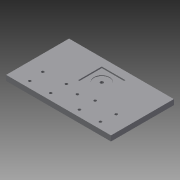
# Autodesk Inventor part: tractor
Saved by Autodesk Inventor 2013 (Build 170138000, 138)
## iProperties
Created: 2012-11-28
Part Number: tractor
Material: Generic
Document SubType Name: Modeling
Designer: Istvan
Density: 1 g/cm^3
Author: Istvan
Autodesk Inventor part; units mm, degrees
ref_plane "YZ Plane" through (0, 0, 0) normal (1, 0, 0) x (0, 1, 0)
ref_plane "XZ Plane" through (0, 0, 0) normal (0, 1, 0) x (-1, 0, 0)
ref_plane "XY Plane" through (0, 0, 0) normal (0, 0, 1) x (1, 0, 0)
sketch "Sketch1" plane through (0, 0, 0) normal (0, 1, 0) x (-1, 0, 0)
  line L0 (0, 0) -> (254, 0)
  line L1 (254, 0) -> (254, 152.4)
  line L2 (254, 152.4) -> (0, 152.4)
  line L3 (0, 152.4) -> (0, 0)
  dimension "d0" = 254
  dimension "d1" = 152.4
  constraints: 8 end point, 2 parallel, 1 horizontal, 1 perpendicular
  measures "d0" distance of L2.end L1.end
  measures "d1" distance of L1.end L0.end
extrude "Extrusion1" add sketch "Sketch1" against normal blind 12.7
sketch "Sketch2" plane through (0, 0, 0) normal (0, 1, 0) x (1, 0, 0)
  line L0 (0, 0) -> (-254, 0) projected
  line L1 (-254, 0) -> (-254, -152.4) projected
  line L2 (0, -152.4) -> (0, 0) projected
  line L3 (-155.575, -19.05) -> (-98.425, -19.05)
  line L4 (-98.425, -19.05) -> (-98.425, -76.2)
  line L5 (-98.425, -76.2) -> (-155.575, -76.2)
  line L6 (-155.575, -76.2) -> (-155.575, -19.05)
  dimension "d4" = 57.15
  dimension "d6" = 57.15
  dimension "d7" = 98.425
  dimension "d8" = 98.425
  dimension "d9" = 19.05
  constraints: 8 end point, 2 parallel, 1 horizontal, 1 perpendicular
  measures "d4" distance of L4.end L5.end
  measures "d6" distance of L3.end L4.end
  measures "d7" distance between parallel lines of L1 L6
  measures "d8" distance between parallel lines of L2 L4
  measures "d9" distance between parallel lines of L0 L3
extrude "Extrusion2" cut sketch "Sketch2" against normal blind 3.175
sketch "Sketch3" plane through (0, -3.175, 0) normal (0, 1, 0) x (1, 0, 0)
  line L0 (-98.425, -76.2) -> (-155.575, -76.2) projected
  line L1 (-98.425, -19.05) -> (-98.425, -76.2) projected
  circle A0 centre (-127, -47.625) radius 19.05
  point P0 (0, 0)
  dimension "d12" = 38.1
  dimension "d13" = 28.575
  dimension "d14" = 28.575
  constraints: 1 centre point
  measures "d12" diameter of A0
  measures "d13" distance from line of L0 A0.centre
  measures "d14" distance from line of L1 A0.centre
extrude "Extrusion3" cut sketch "Sketch3" against normal blind 1.524
sketch "Sketch4" plane through (-127, -4.699, 47.625) normal (0, 1, 0) x (1, 0, 0)
  circle A0 centre (0, 0) radius 19.05 projected
  circle A1 centre (0, 0) radius 3.81
  point P0 (127, 47.625)
  dimension "d17" = 7.62
  constraints: 1 centre point, 1 coincident
  measures "d17" diameter of A1
extrude "Extrusion4" cut sketch "Sketch4" against normal through all contours A1
sketch "Sketch5" plane through (0, -12.7, 0) normal (0, -1, 0) x (1, 0, 0)
  line L0 (0, 0) -> (0, 152.4) projected
  line L1 (0, 152.4) -> (-254, 152.4) projected
  line L2 (-254, 152.4) -> (-254, 0) projected
  circle A0 centre (-127, 47.625) radius 3.81 projected
  point P0 (-38.1, 101.6)
  point P1 (-215.9, 101.6)
  point P2 (-127, 106.68)
  dimension "d20" = 50.8
  dimension "d21" = 38.1
  dimension "d22" = 38.1
  dimension "d30" = 5.08
  constraints: 1 horizontal alignment, 1 vertical alignment
  measures "d20" distance from line of L1 point (-215.9, 101.6)
  measures "d21" distance from line of L2 point (-215.9, 101.6)
  measures "d22" distance from line of L0 point (-38.1, 101.6)
  measures "d30" vertical distance of point (-215.9, 101.6) point (-127, 106.68)
hole "Hole1" at (-38.1, -12.7, 101.6) at (-215.9, -12.7, 101.6) at (-127, -12.7, 106.68) direction (0, 1, 0) diameter 6.35 end through all
sketch "Sketch9" plane through (0, 0, 0) normal (0, 1, 0) x (1, 0, 0)
  circle A0 centre (-127, -106.68) radius 3.175 projected
  circle A1 centre (-161.798, -98.4172) radius 3.175
  circle A2 centre (-161.798, -136.5172) radius 3.175
  circle A3 centre (-212.598, -136.5172) radius 3.175
  circle A4 centre (-92.202, -98.4172) radius 3.175
  circle A5 centre (-92.202, -136.5172) radius 3.175
  circle A6 centre (-41.402, -136.5172) radius 3.175
  dimension "d53" = 69.596
  dimension "d55" = 34.798
  dimension "d56" = 50.8
  dimension "d57" = 38.1
  dimension "d58" = 50.8
  dimension "d59" = 38.1
  constraints: 6 centre point
  measures "d53" distance of A5.centre A2.centre
  measures "d55" horizontal distance of A2.centre A0.centre
  measures "d56" distance of A2.centre A3.centre
  measures "d57" distance of A1.centre A2.centre
  measures "d58" distance of A6.centre A5.centre
  measures "d59" distance of A4.centre A5.centre
hole "Hole4" at (-212.598, 0, 136.5172) at (-161.798, 0, 136.5172) at (-161.798, 0, 98.4172) at (-92.202, 0, 98.4172) at (-92.202, 0, 136.5172) at (-41.402, 0, 136.5172) direction (0, -1, 0) diameter 6.35 end through all
equation "\"d7\" = d8"
equation "\"d22\" = d21"
equation "\"d55\" = 0.5 * d53"
body "Solid1"
